Autodesk Fusion 360 part; units mm, degrees
(part 2 of 2)
sketch "Sketch2" plane through (0, 0, 0) normal (0, 0, 1) x (1, 0, 0)
  line L0 (13, -11) -> (-13, -11)
  line L1 (-15, -9) -> (-15, 9)
  line L2 (-13, 11) -> (13, 11)
  line L3 (15, 9) -> (15, -9)
  arc A0 (-13, 11) -> (-15, 9) centre (-13, 9) ccw
  arc A1 (15, 9) -> (13, 11) centre (13, 9) ccw
  arc A2 (13, -11) -> (15, -9) centre (13, -9) ccw
  arc A3 (-15, -9) -> (-13, -11) centre (-13, -9) ccw
  spline S0 degree 3 poles (4.0459, 5.6596) (3.5021, 5.6173) (3.0747, 5.1464) (3.0512, 4.5644) knots 0 0 0 0 1 1 1 1
  line L4 (3.0512, 4.5644) -> (3.04, 4.0279)
  spline S1 degree 3 poles (3.04, 4.0279) (3.0363, 3.6569) (2.7908, 3.3603) (2.4887, 3.3349) knots 0 0 0 0 1 1 1 1
  spline S2 degree 3 poles (2.4887, 3.3349) (2.4646, 3.334) (2.3592, 3.3316) (2.2502, 3.3275) knots 0 0 0 0 1 1 1 1
  spline S3 degree 3 poles (2.2502, 3.3275) (2.1396, 3.3233) (2.0261, 3.3191) (1.9932, 3.3163) knots 0 0 0 0 1 1 1 1
  spline S4 degree 3 poles (1.9932, 3.3163) (1.6944, 3.2927) (1.4246, 3.1392) (1.2406, 2.8953) knots 0 0 0 0 1 1 1 1
  spline S5 degree 3 poles (1.2406, 2.8953) (1.1016, 2.7203) (1.0144, 2.5064) (0.991, 2.2806) knots 0 0 0 0 1 1 1 1
  spline S6 degree 3 poles (0.991, 2.2806) (0.9833, 2.1986) (0.9814, 2.1189) (0.9873, 2.0459) knots 0 0 0 0 1 1 1 1
  spline S7 degree 3 poles (0.9873, 2.0459) (0.9878, 2.0323) (0.9902, 1.9387) (0.991, 1.8522) knots 0 0 0 0 1 1 1 1
  spline S8 degree 2 poles (0.991, 1.8522) (0.9918, 1.7658) (0.991, 1.6846) knots 0 0 0 1 1 1
  spline S9 degree 3 poles (0.991, 1.6846) (0.9873, 1.3122) (0.7435, 1.0171) (0.4322, 0.9916) knots 0 0 0 0 1 1 1 1
  line L5 (0.4322, 0.9916) -> (-0.067, 0.9544)
  spline S10 degree 3 poles (-0.067, 0.9544) (-0.567, 0.9157) (-0.9691, 0.5308) (-1.0431, 0.0267) knots 0 0 0 0 1 1 1 1
  spline S11 degree 3 poles (-1.0431, 0.0267) (-1.0554, -0.0509) (-1.0599, -0.2159) (-1.0617, -0.2489) knots 0 0 0 0 1 1 1 1
  line L6 (-1.0617, -0.2489) -> (-1.0729, -0.7295)
  spline S12 degree 3 poles (-1.0729, -0.7295) (-1.0716, -1.0904) (-1.3155, -1.3812) (-1.6429, -1.4113) knots 0 0 0 0 1 1 1 1
  spline S13 degree 3 poles (-1.6429, -1.4113) (-1.6727, -1.4113) (-1.7757, -1.4076) (-1.8813, -1.4076) knots 0 0 0 0 1 1 1 1
  spline S14 degree 3 poles (-1.8813, -1.4076) (-2.0004, -1.4076) (-2.0851, -1.4106) (-2.1384, -1.4187) knots 0 0 0 0 1 1 1 1
  spline S15 degree 3 poles (-2.1384, -1.4187) (-2.5218, -1.4731) (-2.8335, -1.6981) (-2.9952, -2.026) knots 0 0 0 0 1 1 1 1
  spline S16 degree 3 poles (-2.9952, -2.026) (-3.1043, -2.2305) (-3.153, -2.4605) (-3.1331, -2.6891) knots 0 0 0 0 1 1 1 1
  spline S17 degree 2 poles (-3.1331, -2.6891) (-3.1319, -2.7171) (-3.1219, -3.0766) knots 0 0 0 1 1 1
  spline S18 degree 3 poles (-3.1219, -3.0766) (-3.1164, -3.4412) (-3.3659, -3.729) (-3.6993, -3.7546) knots 0 0 0 0 1 1 1 1
  spline S19 degree 2 poles (-3.6993, -3.7546) (-3.9764, -3.766) (-4.5674, -3.7807) knots 0 0 0 1 1 1
  spline S20 degree 3 poles (-4.5674, -3.7807) (-4.8976, -3.777) (-5.1727, -3.4978) (-5.2044, -3.1287) knots 0 0 0 0 1 1 1 1
  line L7 (-5.2044, -3.1287) -> (-5.2156, -2.9574)
  spline S21 degree 3 poles (-5.2156, -2.9574) (-5.219, -2.9233) (-5.217, -2.8652) (-5.2156, -2.8083) knots 0 0 0 0 1 1 1 1
  spline S22 degree 3 poles (-5.2156, -2.8083) (-5.2156, -2.7383) (-5.2153, -2.6722) (-5.2193, -2.6183) knots 0 0 0 0 1 1 1 1
  spline S23 degree 3 poles (-5.2193, -2.6183) (-5.251, -2.2243) (-5.4718, -1.8745) (-5.8005, -1.687) knots 0 0 0 0 1 1 1 1
  spline S24 degree 3 poles (-5.8005, -1.687) (-5.9946, -1.5677) (-6.223, -1.5137) (-6.4338, -1.5305) knots 0 0 0 0 1 1 1 1
  line L8 (-6.4338, -1.5305) -> (-6.4674, -1.5342)
  spline S25 degree 3 poles (-6.4674, -1.5342) (-6.4962, -1.5355) (-6.5295, -1.536) (-6.553, -1.538) knots 0 0 0 0 1 1 1 1
  line L9 (-6.553, -1.538) -> (-6.7877, -1.5342)
  spline S26 degree 3 poles (-6.7877, -1.5342) (-7.1178, -1.5324) (-7.3917, -1.2536) (-7.4248, -0.8823) knots 0 0 0 0 1 1 1 1
  line L10 (-7.4248, -0.8823) -> (-7.4658, -0.4017)
  spline S27 degree 3 poles (-7.4658, -0.4017) (-7.465, -0.3887) (-7.4643, -0.374) (-7.4658, -0.357) knots 0 0 0 0 1 1 1 1
  spline S28 degree 3 poles (-7.4658, -0.357) (-7.5196, 0.2738) (-8.055, 0.7631) (-8.6542, 0.7159) knots 0 0 0 0 1 1 1 1
  spline S29 degree 3 poles (-8.6542, 0.7159) (-8.9328, 0.6945) (-9.1922, 0.562) (-9.3769, 0.3434) knots 0 0 0 0 1 1 1 1
  spline S30 degree 3 poles (-9.3769, 0.3434) (-9.5782, 0.1068) (-9.6758, -0.2119) (-9.6489, -0.5321) knots 0 0 0 0 1 1 1 1
  spline S31 degree 3 poles (-9.6489, -0.5321) (-9.6, -1.1036) (-9.1563, -1.5632) (-8.6095, -1.6013) knots 0 0 0 0 1 1 1 1
  line L11 (-8.6095, -1.6013) -> (-8.1028, -1.6236)
  spline S32 degree 3 poles (-8.1028, -1.6236) (-7.7639, -1.6346) (-7.4867, -1.9029) (-7.4583, -2.2458) knots 0 0 0 0 1 1 1 1
  line L12 (-7.4583, -2.2458) -> (-7.4397, -2.6481)
  spline S33 degree 3 poles (-7.4397, -2.6481) (-7.4378, -2.6968) (-7.4361, -2.7355) (-7.4322, -2.7785) knots 0 0 0 0 1 1 1 1
  spline S34 degree 3 poles (-7.4322, -2.7785) (-7.4053, -3.0916) (-7.2625, -3.376) (-7.0336, -3.5758) knots 0 0 0 0 1 1 1 1
  spline S35 degree 3 poles (-7.0336, -3.5758) (-6.8658, -3.7313) (-6.6644, -3.8268) (-6.4487, -3.8552) knots 0 0 0 0 1 1 1 1
  spline S36 degree 3 poles (-6.4487, -3.8552) (-6.3703, -3.867) (-6.2961, -3.8702) (-6.214, -3.8664) knots 0 0 0 0 1 1 1 1
  spline S37 degree 2 poles (-6.214, -3.8664) (-6.1486, -3.8664) (-5.8862, -3.8664) knots 0 0 0 1 1 1
  spline S38 degree 3 poles (-5.8862, -3.8664) (-5.5473, -3.8773) (-5.2676, -4.1511) (-5.2379, -4.4997) knots 0 0 0 0 1 1 1 1
  line L13 (-5.2379, -4.4997) -> (-5.1932, -5.0362)
  spline S39 degree 3 poles (-5.1932, -5.0362) (-5.1463, -5.5846) (-4.7415, -6.033) (-4.2283, -6.1016) knots 0 0 0 0 1 1 1 1
  spline S40 degree 3 poles (-4.2283, -6.1016) (-4.1746, -6.1095) (-4.1195, -6.1128) (-4.0682, -6.1128) knots 0 0 0 0 1 1 1 1
  spline S41 degree 3 poles (-4.0682, -6.1128) (-4.0434, -6.1128) (-4.0177, -6.1141) (-3.9936, -6.1128) knots 0 0 0 0 1 1 1 1
  spline S42 degree 3 poles (-3.9936, -6.1128) (-3.4506, -6.0698) (-3.0247, -5.5991) (-3.0027, -5.0175) knots 0 0 0 0 1 1 1 1
  line L14 (-3.0027, -5.0175) -> (-2.9915, -4.4811)
  spline S43 degree 3 poles (-2.9915, -4.4811) (-2.9878, -4.1081) (-2.742, -3.8123) (-2.4364, -3.7881) knots 0 0 0 0 1 1 1 1
  spline S44 degree 2 poles (-2.4364, -3.7881) (-2.3291, -3.7855) (-2.2129, -3.7807) knots 0 0 0 1 1 1
  spline S45 degree 3 poles (-2.2129, -3.7807) (-2.0967, -3.7759) (-1.9752, -3.772) (-1.9446, -3.7695) knots 0 0 0 0 1 1 1 1
  spline S46 degree 3 poles (-1.9446, -3.7695) (-1.6459, -3.7467) (-1.3768, -3.5944) (-1.1921, -3.3523) knots 0 0 0 0 1 1 1 1
  spline S47 degree 3 poles (-1.1921, -3.3523) (-1.0505, -3.1759) (-0.9616, -2.9604) (-0.9387, -2.7338) knots 0 0 0 0 1 1 1 1
  spline S48 degree 3 poles (-0.9387, -2.7338) (-0.931, -2.6518) (-0.9291, -2.5728) (-0.935, -2.4991) knots 0 0 0 0 1 1 1 1
  spline S49 degree 2 poles (-0.935, -2.4991) (-0.935, -2.4638) (-0.9387, -2.1378) knots 0 0 0 1 1 1
  spline S50 degree 3 poles (-0.9387, -2.1378) (-0.9351, -1.7654) (-0.6942, -1.469) (-0.3837, -1.4448) knots 0 0 0 0 1 1 1 1
  line L15 (-0.3837, -1.4448) -> (0.1155, -1.4076)
  spline S51 degree 3 poles (0.1155, -1.4076) (0.6107, -1.3673) (1.018, -0.9888) (1.1065, -0.4911) knots 0 0 0 0 1 1 1 1
  spline S52 degree 3 poles (1.1065, -0.4911) (1.1072, -0.4861) (1.1115, -0.4749) (1.114, -0.4427) knots 0 0 0 0 1 1 1 1
  spline S53 degree 3 poles (1.114, -0.4427) (1.1164, -0.4104) (1.1204, -0.3544) (1.1251, -0.2452) knots 0 0 0 0 1 1 1 1
  line L16 (1.1251, -0.2452) -> (1.1214, 0.2801)
  spline S54 degree 3 poles (1.1214, 0.2801) (1.1196, 0.6442) (1.3699, 0.9362) (1.7026, 0.9618) knots 0 0 0 0 1 1 1 1
  line L17 (1.7026, 0.9618) -> (1.8032, 0.9693)
  line L18 (1.8032, 0.9693) -> (1.8255, 0.9693)
  spline S55 degree 3 poles (1.8255, 0.9693) (1.8551, 0.9693) (1.8984, 0.9656) (1.9447, 0.9656) knots 0 0 0 0 1 1 1 1
  spline S56 degree 3 poles (1.9447, 0.9656) (2.0328, 0.9617) (2.1257, 0.9614) (2.1757, 0.9656) knots 0 0 0 0 1 1 1 1
  spline S57 degree 3 poles (2.1757, 0.9656) (2.5513, 0.9954) (2.8768, 1.2246) (3.0475, 1.5728) knots 0 0 0 0 1 1 1 1
  spline S58 degree 3 poles (3.0475, 1.5728) (3.1445, 1.7584) (3.1892, 1.978) (3.1816, 2.2285) knots 0 0 0 0 1 1 1 1
  spline S59 degree 2 poles (3.1816, 2.2285) (3.1778, 2.3719) (3.1704, 2.6234) knots 0 0 0 1 1 1
  spline S60 degree 3 poles (3.1704, 2.6234) (3.1668, 2.9873) (3.4171, 3.2782) (3.7479, 3.3051) knots 0 0 0 0 1 1 1 1
  spline S61 degree 2 poles (3.7479, 3.3051) (4.4296, 3.3308) (4.6159, 3.3275) knots 0 0 0 1 1 1
  spline S62 degree 3 poles (4.6196, 3.3275) (4.9499, 3.3239) (5.2256, 3.0454) (5.2567, 2.6867) knots 0 0 0 0 1 1 1 1
  spline S63 degree 3 poles (5.2567, 2.6867) (5.2568, 2.6344) (5.2634, 2.2542) (5.2716, 2.1652) knots 0 0 0 0 1 1 1 1
  spline S64 degree 3 poles (5.2716, 2.1652) (5.3046, 1.772) (5.5193, 1.4251) (5.8453, 1.2375) knots 0 0 0 0 1 1 1 1
  spline S65 degree 3 poles (5.8453, 1.2375) (6.0161, 1.1303) (6.2078, 1.0736) (6.4041, 1.0736) knots 0 0 0 0 1 1 1 1
  spline S66 degree 3 poles (6.4041, 1.0736) (6.4302, 1.0736) (6.4563, 1.0749) (6.4786, 1.0773) knots 0 0 0 0 1 1 1 1
  spline S67 degree 3 poles (6.4786, 1.0773) (6.5101, 1.078) (6.838, 1.081) (6.84, 1.081) knots 0 0 0 0 1 1 1 1
  spline S68 degree 3 poles (6.84, 1.081) (7.1717, 1.0774) (7.4446, 0.799) (7.477, 0.4291) knots 0 0 0 0 1 1 1 1
  spline S69 degree 3 poles (7.477, 0.4291) (7.4776, 0.422) (7.5175, -0.0822) (7.518, -0.0962) knots 0 0 0 0 1 1 1 1
  spline S70 degree 3 poles (7.518, -0.0962) (7.5732, -0.7268) (8.1044, -1.219) (8.7065, -1.1691) knots 0 0 0 0 1 1 1 1
  spline S71 degree 3 poles (8.7065, -1.1691) (8.9852, -1.1477) (9.2401, -1.0144) (9.4255, -0.7966) knots 0 0 0 0 1 1 1 1
  spline S72 degree 3 poles (9.4255, -0.7966) (9.6268, -0.5593) (9.7281, -0.2393) (9.7012, 0.0789) knots 0 0 0 0 1 1 1 1
  spline S73 degree 3 poles (9.7012, 0.0789) (9.6521, 0.6503) (9.2049, 1.1107) (8.658, 1.1481) knots 0 0 0 0 1 1 1 1
  line L19 (8.658, 1.1481) -> (8.1588, 1.1705)
  spline S74 degree 3 poles (8.1588, 1.1705) (7.8184, 1.1814) (7.5389, 1.4527) (7.5106, 1.7963) knots 0 0 0 0 1 1 1 1
  spline S75 degree 3 poles (7.5106, 1.7963) (7.5083, 1.8506) (7.4867, 2.2523) (7.4808, 2.3216) knots 0 0 0 0 1 1 1 1
  line L20 (7.4808, 2.3216) -> (7.4808, 2.3253)
  spline S76 degree 3 poles (7.4808, 2.3253) (7.4552, 2.6352) (7.3123, 2.9185) (7.0859, 3.1189) knots 0 0 0 0 1 1 1 1
  spline S77 degree 3 poles (7.0859, 3.1189) (6.9172, 3.2757) (6.7121, 3.3736) (6.4935, 3.402) knots 0 0 0 0 1 1 1 1
  spline S78 degree 3 poles (6.4935, 3.402) (6.4172, 3.4138) (6.3463, 3.419) (6.2626, 3.4132) knots 0 0 0 0 1 1 1 1
  spline S79 degree 3 poles (6.2626, 3.4132) (6.1965, 3.4132) (5.9468, 3.4168) (5.9384, 3.4169) knots 0 0 0 0 1 1 1 1
  line L21 (5.9384, 3.4169) -> (5.9347, 3.4169)
  spline S80 degree 3 poles (5.9347, 3.4169) (5.5958, 3.4294) (5.3192, 3.6983) (5.2902, 4.0465) knots 0 0 0 0 1 1 1 1
  line L22 (5.2902, 4.0465) -> (5.2418, 4.583)
  spline S81 degree 3 poles (5.2418, 4.583) (5.1943, 5.1308) (4.7895, 5.5805) (4.2769, 5.6485) knots 0 0 0 0 1 1 1 1
  spline S82 degree 3 poles (4.2769, 5.6485) (4.1971, 5.6602) (4.1232, 5.6656) (4.0459, 5.6596) knots 0 0 0 0 1 1 1 1
  spline S83 degree 3 poles (2.0453, 7.8949) (1.4432, 7.8459) (0.9839, 7.3052) (0.9761, 6.6394) knots 0 0 0 0 1 1 1 1
  line L23 (0.9761, 6.6394) -> (0.9761, 6.0434)
  spline S84 degree 3 poles (0.9761, 6.0434) (0.9797, 5.6358) (0.7138, 5.3125) (0.3651, 5.2796) knots 0 0 0 0 1 1 1 1
  line L24 (0.3651, 5.2796) -> (0.2608, 5.2796)
  spline S85 degree 3 poles (0.2608, 5.2796) (-0.076, 5.2796) (-0.1303, 5.2736) (-0.149, 5.2722) knots 0 0 0 0 1 1 1 1
  spline S86 degree 3 poles (-0.149, 5.2722) (-0.5528, 5.2397) (-0.9047, 4.9814) (-1.0878, 4.5904) knots 0 0 0 0 1 1 1 1
  spline S87 degree 3 poles (-1.0878, 4.5904) (-1.2021, 4.3647) (-1.2542, 4.1071) (-1.2331, 3.8491) knots 0 0 0 0 1 1 1 1
  spline S88 degree 3 poles (-1.2331, 3.8491) (-1.2325, 3.8453) (-1.2309, 3.8092) (-1.2294, 3.7671) knots 0 0 0 0 1 1 1 1
  spline S89 degree 3 poles (-1.2294, 3.7671) (-1.2279, 3.725) (-1.2232, 3.6732) (-1.2219, 3.6218) knots 0 0 0 0 1 1 1 1
  spline S90 degree 2 poles (-1.2219, 3.6218) (-1.2193, 3.5191) (-1.2182, 3.4206) knots 0 0 0 1 1 1
  spline S91 degree 3 poles (-1.2182, 3.4206) (-1.2146, 3.0094) (-1.4806, 2.6825) (-1.8329, 2.6532) knots 0 0 0 0 1 1 1 1
  spline S92 degree 3 poles (-1.8329, 2.6532) (-2.1688, 2.6347) (-2.7558, 2.6272) (-2.7605, 2.6271) knots 0 0 0 0 1 1 1 1
  spline S93 degree 3 poles (-2.7605, 2.6271) (-3.1154, 2.6313) (-3.4103, 2.9423) (-3.4423, 3.3461) knots 0 0 0 0 1 1 1 1
  spline S94 degree 3 poles (-3.4423, 3.3461) (-3.4432, 3.3696) (-3.4466, 3.4939) (-3.4497, 3.6218) knots 0 0 0 0 1 1 1 1
  spline S95 degree 3 poles (-3.4497, 3.6218) (-3.4528, 3.7497) (-3.4569, 3.8808) (-3.4609, 3.931) knots 0 0 0 0 1 1 1 1
  spline S96 degree 3 poles (-3.4609, 3.931) (-3.4968, 4.3707) (-3.729, 4.7587) (-4.0793, 4.9667) knots 0 0 0 0 1 1 1 1
  spline S97 degree 3 poles (-4.0793, 4.9667) (-4.2616, 5.0859) (-4.4689, 5.1492) (-4.6791, 5.1492) knots 0 0 0 0 1 1 1 1
  spline S98 degree 3 poles (-4.6791, 5.1492) (-4.7098, 5.1492) (-4.7405, 5.1474) (-4.7648, 5.1455) knots 0 0 0 0 1 1 1 1
  spline S99 degree 3 poles (-4.7648, 5.1455) (-4.7791, 5.1448) (-4.8755, 5.1461) (-4.966, 5.1455) knots 0 0 0 0 1 1 1 1
  spline S100 degree 3 poles (-4.966, 5.1455) (-5.0113, 5.1452) (-5.056, 5.1421) (-5.0889, 5.1418) knots 0 0 0 0 1 1 1 1
  spline S101 degree 3 poles (-5.0889, 5.1418) (-5.1054, 5.1417) (-5.1203, 5.1419) (-5.1299, 5.1418) knots 0 0 0 0 1 1 1 1
  spline S102 degree 3 poles (-5.1299, 5.1418) (-5.1347, 5.1417) (-5.1384, 5.1419) (-5.1411, 5.1418) knots 0 0 0 0 1 1 1 1
  line L25 (-5.1411, 5.1418) -> (-5.1448, 5.1418)
  spline S103 degree 3 poles (-5.1448, 5.1418) (-5.4952, 5.1453) (-5.8088, 5.5001) (-5.8415, 5.9167) knots 0 0 0 0 1 1 1 1
  spline S104 degree 2 poles (-5.8415, 5.9167) (-5.8525, 6.059) (-5.8638, 6.2036) knots 0 0 0 1 1 1
  spline S105 degree 3 poles (-5.8638, 6.2036) (-5.8695, 6.2759) (-5.8781, 6.3486) (-5.8825, 6.4047) knots 0 0 0 0 1 1 1 1
  spline S106 degree 3 poles (-5.8825, 6.4047) (-5.8846, 6.4328) (-5.8849, 6.4543) (-5.8862, 6.4718) knots 0 0 0 0 1 1 1 1
  spline S107 degree 3 poles (-5.8862, 6.4718) (-5.8875, 6.4893) (-5.8899, 6.5019) (-5.8899, 6.5016) knots 0 0 0 0 1 1 1 1
  line L26 (-5.8899, 6.5016) -> (-5.8899, 6.5053)
  spline S108 degree 3 poles (-5.8899, 6.5053) (-5.9446, 7.1774) (-6.4653, 7.7049) (-7.0783, 7.7049) knots 0 0 0 0 1 1 1 1
  spline S109 degree 3 poles (-7.0783, 7.7049) (-7.1077, 7.7049) (-7.1364, 7.7069) (-7.1677, 7.7049) knots 0 0 0 0 1 1 1 1
  spline S110 degree 3 poles (-7.1677, 7.7049) (-7.4614, 7.6808) (-7.733, 7.5349) (-7.9315, 7.2988) knots 0 0 0 0 1 1 1 1
  spline S111 degree 3 poles (-7.9315, 7.2988) (-8.1548, 7.034) (-8.2617, 6.6735) (-8.2332, 6.3116) knots 0 0 0 0 1 1 1 1
  spline S112 degree 3 poles (-8.2332, 6.3116) (-8.1807, 5.673) (-7.7048, 5.1609) (-7.1156, 5.1194) knots 0 0 0 0 1 1 1 1
  line L27 (-7.1156, 5.1194) -> (-6.5754, 5.0934)
  spline S113 degree 3 poles (-6.5754, 5.0934) (-6.2178, 5.0815) (-5.8993, 4.7373) (-5.8676, 4.352) knots 0 0 0 0 1 1 1 1
  spline S114 degree 3 poles (-5.8676, 4.352) (-5.8661, 4.2932) (-5.8402, 3.832) (-5.834, 3.7597) knots 0 0 0 0 1 1 1 1
  spline S115 degree 3 poles (-5.834, 3.7597) (-5.8055, 3.4129) (-5.6588, 3.0933) (-5.4168, 2.8693) knots 0 0 0 0 1 1 1 1
  spline S116 degree 3 poles (-5.4168, 2.8693) (-5.2351, 2.6943) (-5.0153, 2.5858) (-4.7834, 2.5526) knots 0 0 0 0 1 1 1 1
  spline S117 degree 3 poles (-4.7834, 2.5526) (-4.7472, 2.5463) (-4.7035, 2.5452) (-4.6456, 2.5452) knots 0 0 0 0 1 1 1 1
  spline S118 degree 3 poles (-4.6456, 2.5452) (-4.6038, 2.5452) (-4.5356, 2.5432) (-4.4929, 2.5452) knots 0 0 0 0 1 1 1 1
  line L28 (-4.4929, 2.5452) -> (-4.1799, 2.5414)
  spline S119 degree 3 poles (-4.1799, 2.5414) (-3.8186, 2.5267) (-3.5196, 2.2229) (-3.487, 1.8299) knots 0 0 0 0 1 1 1 1
  line L29 (-3.487, 1.8299) -> (-3.4385, 1.2263)
  spline S120 degree 3 poles (-3.4385, 1.2263) (-3.3876, 0.615) (-2.9511, 0.1141) (-2.3991, 0.0379) knots 0 0 0 0 1 1 1 1
  spline S121 degree 3 poles (-2.3991, 0.0379) (-2.3406, 0.028) (-2.2843, 0.0267) (-2.2315, 0.0267) knots 0 0 0 0 1 1 1 1
  spline S122 degree 3 poles (-2.2315, 0.0267) (-2.2044, 0.0267) (-2.1774, 0.0247) (-2.1495, 0.0267) knots 0 0 0 0 1 1 1 1
  spline S123 degree 3 poles (-2.1495, 0.0267) (-1.5651, 0.0743) (-1.1082, 0.5978) (-1.0803, 1.245) knots 0 0 0 0 1 1 1 1
  line L30 (-1.0803, 1.245) -> (-1.0803, 1.2487)
  line L31 (-1.0803, 1.2487) -> (-1.0691, 1.8522)
  spline S124 degree 3 poles (-1.0691, 1.8522) (-1.0641, 2.2718) (-0.8083, 2.6015) (-0.4843, 2.6271) knots 0 0 0 0 1 1 1 1
  spline S125 degree 3 poles (-0.4843, 2.6271) (-0.4617, 2.6285) (-0.3418, 2.633) (-0.2235, 2.6383) knots 0 0 0 0 1 1 1 1
  spline S126 degree 3 poles (-0.2235, 2.6383) (-0.1051, 2.6436) (0.0114, 2.6499) (0.0448, 2.6532) knots 0 0 0 0 1 1 1 1
  spline S127 degree 3 poles (0.0448, 2.6532) (0.3683, 2.6796) (0.6563, 2.8462) (0.8569, 3.1189) knots 0 0 0 0 1 1 1 1
  spline S128 degree 3 poles (0.8569, 3.1189) (1.0071, 3.3149) (1.1019, 3.5507) (1.1251, 3.8006) knots 0 0 0 0 1 1 1 1
  spline S129 degree 3 poles (1.1251, 3.8006) (1.1349, 3.8932) (1.1347, 3.9848) (1.1289, 4.0689) knots 0 0 0 0 1 1 1 1
  spline S130 degree 3 poles (1.1289, 4.0689) (1.1281, 4.0856) (1.1263, 4.1922) (1.1251, 4.2887) knots 0 0 0 0 1 1 1 1
  spline S131 degree 2 poles (1.1251, 4.2887) (1.1239, 4.3852) (1.1251, 4.4749) knots 0 0 0 1 1 1
  spline S132 degree 3 poles (1.1251, 4.4749) (1.1308, 4.8938) (1.3893, 5.225) (1.7212, 5.2536) knots 0 0 0 0 1 1 1 1
  line L32 (1.7212, 5.2536) -> (2.254, 5.2945)
  spline S133 degree 3 poles (2.254, 5.2945) (2.8198, 5.3406) (3.2647, 5.8229) (3.3194, 6.4345) knots 0 0 0 0 1 1 1 1
  spline S134 degree 3 poles (3.3194, 6.4345) (3.3292, 6.5215) (3.331, 6.6109) (3.3232, 6.699) knots 0 0 0 0 1 1 1 1
  spline S135 degree 3 poles (3.3232, 6.699) (3.2647, 7.4027) (2.6924, 7.9493) (2.0453, 7.8949) knots 0 0 0 0 1 1 1 1
  spline S136 degree 3 poles (-8.8405, 5.2573) (-9.3781, 5.2128) (-9.8036, 4.7297) (-9.8277, 4.1359) knots 0 0 0 0 1 1 1 1
  line L33 (-9.8277, 4.1359) -> (-9.8389, 3.5808)
  spline S137 degree 3 poles (-9.8389, 3.5808) (-9.8426, 3.1977) (-10.0794, 2.8977) (-10.3754, 2.873) knots 0 0 0 0 1 1 1 1
  spline S138 degree 3 poles (-10.3754, 2.873) (-10.3996, 2.8722) (-10.5027, 2.8698) (-10.6101, 2.8655) knots 0 0 0 0 1 1 1 1
  spline S139 degree 3 poles (-10.6101, 2.8655) (-10.7192, 2.8612) (-10.8305, 2.8538) (-10.8634, 2.8506) knots 0 0 0 0 1 1 1 1
  spline S140 degree 3 poles (-10.8634, 2.8506) (-11.16, 2.8255) (-11.4279, 2.6707) (-11.6122, 2.4222) knots 0 0 0 0 1 1 1 1
  spline S141 degree 3 poles (-11.6122, 2.4222) (-11.7505, 2.2413) (-11.8367, 2.0206) (-11.8581, 1.7889) knots 0 0 0 0 1 1 1 1
  spline S142 degree 3 poles (-11.8581, 1.7889) (-11.868, 1.7102) (-11.8676, 1.627) (-11.8618, 1.543) knots 0 0 0 0 1 1 1 1
  spline S143 degree 3 poles (-11.8618, 1.543) (-11.8087, 0.896) (-11.2812, 0.3954) (-10.6808, 0.444) knots 0 0 0 0 1 1 1 1
  spline S144 degree 3 poles (-10.6808, 0.444) (-10.3068, 0.4739) (-9.9812, 0.7117) (-9.8128, 1.0699) knots 0 0 0 0 1 1 1 1
  spline S145 degree 3 poles (-9.8128, 1.0699) (-9.7066, 1.2783) (-9.6601, 1.5123) (-9.6787, 1.7479) knots 0 0 0 0 1 1 1 1
  spline S146 degree 3 poles (-9.6787, 1.7479) (-9.6795, 1.7614) (-9.684, 1.8653) (-9.6861, 1.9603) knots 0 0 0 0 1 1 1 1
  spline S147 degree 2 poles (-9.6861, 1.9603) (-9.6883, 2.0552) (-9.6899, 2.1428) knots 0 0 0 1 1 1
  spline S148 degree 3 poles (-9.6899, 2.1428) (-9.6936, 2.5176) (-9.4519, 2.817) (-9.1273, 2.8432) knots 0 0 0 0 1 1 1 1
  spline S149 degree 2 poles (-9.1273, 2.8432) (-8.6249, 2.8668) (-8.2742, 2.8655) knots 0 0 0 1 1 1
  spline S150 degree 3 poles (-8.2742, 2.8655) (-8.2732, 2.8655) (-8.2715, 2.8656) (-8.2705, 2.8655) knots 0 0 0 0 1 1 1 1
  spline S151 degree 3 poles (-8.2705, 2.8655) (-8.1132, 2.8626) (-7.9448, 2.7694) (-7.8122, 2.6271) knots 0 0 0 0 1 1 1 1
  spline S152 degree 3 poles (-7.8122, 2.6271) (-7.6788, 2.4839) (-7.5815, 2.292) (-7.5663, 2.1093) knots 0 0 0 0 1 1 1 1
  spline S153 degree 3 poles (-7.5663, 2.1093) (-7.5657, 2.0853) (-7.5653, 1.9752) (-7.5626, 1.8597) knots 0 0 0 0 1 1 1 1
  spline S154 degree 3 poles (-7.5626, 1.8597) (-7.5599, 1.7425) (-7.5556, 1.623) (-7.5515, 1.5765) knots 0 0 0 0 1 1 1 1
  spline S155 degree 3 poles (-7.5515, 1.5765) (-7.5186, 1.1754) (-7.3036, 0.8203) (-6.9815, 0.6265) knots 0 0 0 0 1 1 1 1
  spline S156 degree 3 poles (-6.9815, 0.6265) (-6.8132, 0.5172) (-6.6178, 0.4589) (-6.4226, 0.4589) knots 0 0 0 0 1 1 1 1
  spline S157 degree 3 poles (-6.4226, 0.4589) (-6.3954, 0.4589) (-6.3703, 0.4602) (-6.3481, 0.4626) knots 0 0 0 0 1 1 1 1
  spline S158 degree 3 poles (-6.3481, 0.4626) (-6.3159, 0.4632) (-6.0045, 0.4663) (-5.9979, 0.4663) knots 0 0 0 0 1 1 1 1
  spline S159 degree 3 poles (-5.9979, 0.4663) (-5.6758, 0.4627) (-5.407, 0.1757) (-5.3758, -0.2042) knots 0 0 0 0 1 1 1 1
  spline S160 degree 3 poles (-5.3758, -0.2042) (-5.3755, -0.2078) (-5.3634, -0.3287) (-5.3534, -0.4576) knots 0 0 0 0 1 1 1 1
  spline S161 degree 3 poles (-5.3534, -0.4576) (-5.3484, -0.5229) (-5.3462, -0.5915) (-5.3423, -0.6438) knots 0 0 0 0 1 1 1 1
  spline S162 degree 3 poles (-5.3423, -0.6438) (-5.3383, -0.6962) (-5.335, -0.7347) (-5.3348, -0.7407) knots 0 0 0 0 1 1 1 1
  line L34 (-5.3348, -0.7407) -> (-5.3348, -0.7444)
  spline S163 degree 3 poles (-5.3348, -0.7444) (-5.2803, -1.3912) (-4.7562, -1.8927) (-4.1538, -1.8434) knots 0 0 0 0 1 1 1 1
  spline S164 degree 3 poles (-4.1538, -1.8434) (-3.553, -1.7943) (-3.1129, -1.2185) (-3.1666, -0.5656) knots 0 0 0 0 1 1 1 1
  spline S165 degree 3 poles (-3.1666, -0.5656) (-3.2141, 0.0208) (-3.654, 0.4908) (-4.1985, 0.5297) knots 0 0 0 0 1 1 1 1
  line L35 (-4.1985, 0.5297) -> (-4.694, 0.5558)
  spline S166 degree 3 poles (-4.694, 0.5558) (-5.0221, 0.5666) (-5.2956, 0.8434) (-5.3274, 1.1928) knots 0 0 0 0 1 1 1 1
  spline S167 degree 3 poles (-5.3274, 1.1928) (-5.3288, 1.2464) (-5.3521, 1.6713) (-5.3572, 1.7367) knots 0 0 0 0 1 1 1 1
  spline S168 degree 3 poles (-5.3572, 1.7367) (-5.3841, 2.0548) (-5.5222, 2.346) (-5.7446, 2.5526) knots 0 0 0 0 1 1 1 1
  spline S169 degree 3 poles (-5.7446, 2.5526) (-5.9109, 2.7133) (-6.113, 2.8165) (-6.3258, 2.8469) knots 0 0 0 0 1 1 1 1
  line L36 (-6.3258, 2.8469) -> (-6.3295, 2.8469)
  spline S170 degree 3 poles (-6.3295, 2.8469) (-6.4068, 2.8581) (-6.4908, 2.8599) (-6.5568, 2.8544) knots 0 0 0 0 1 1 1 1
  line L37 (-6.5568, 2.8544) -> (-6.5866, 2.8544)
  spline S171 degree 3 poles (-6.5866, 2.8544) (-6.672, 2.8544) (-6.8763, 2.8581) (-6.8846, 2.8581) knots 0 0 0 0 1 1 1 1
  line L38 (-6.8846, 2.8581) -> (-6.8883, 2.8581)
  spline S172 degree 3 poles (-6.8883, 2.8581) (-7.0501, 2.8654) (-7.2235, 2.9601) (-7.3577, 3.1002) knots 0 0 0 0 1 1 1 1
  spline S173 degree 3 poles (-7.3577, 3.1002) (-7.4928, 3.2413) (-7.5889, 3.4252) (-7.6036, 3.6032) knots 0 0 0 0 1 1 1 1
  line L39 (-7.6036, 3.6032) -> (-7.6483, 4.1546)
  spline S174 degree 3 poles (-7.6483, 4.1546) (-7.6938, 4.7167) (-8.0972, 5.1797) (-8.6095, 5.2498) knots 0 0 0 0 1 1 1 1
  spline S175 degree 3 poles (-8.6095, 5.2498) (-8.6609, 5.2578) (-8.7092, 5.2573) (-8.7585, 5.2573) knots 0 0 0 0 1 1 1 1
  spline S176 degree 3 poles (-8.7585, 5.2573) (-8.7841, 5.2573) (-8.8115, 5.2593) (-8.8405, 5.2573) knots 0 0 0 0 1 1 1 1
  spline S177 degree 3 poles (2.2689, -0.8078) (2.2428, -0.8078) (2.2159, -0.8102) (2.1906, -0.8115) knots 0 0 0 0 1 1 1 1
  spline S178 degree 3 poles (2.1906, -0.8115) (1.653, -0.856) (1.2349, -1.3378) (1.2108, -1.9329) knots 0 0 0 0 1 1 1 1
  line L40 (1.2108, -1.9329) -> (1.1997, -2.4879)
  spline S179 degree 3 poles (1.1997, -2.4879) (1.196, -2.8718) (0.956, -3.1717) (0.6595, -3.1958) knots 0 0 0 0 1 1 1 1
  spline S180 degree 3 poles (0.6595, -3.1958) (0.6115, -3.1979) (0.2381, -3.2171) (0.1789, -3.2219) knots 0 0 0 0 1 1 1 1
  spline S181 degree 3 poles (0.1789, -3.2219) (-0.1188, -3.2449) (-0.3855, -3.3996) (-0.57, -3.6503) knots 0 0 0 0 1 1 1 1
  spline S182 degree 3 poles (-0.57, -3.6503) (-0.7061, -3.83) (-0.7932, -4.0471) (-0.8158, -4.2762) knots 0 0 0 0 1 1 1 1
  spline S183 degree 3 poles (-0.8158, -4.2762) (-0.8256, -4.3615) (-0.8275, -4.447) (-0.8195, -4.5258) knots 0 0 0 0 1 1 1 1
  spline S184 degree 3 poles (-0.8195, -4.5258) (-0.819, -4.5436) (-0.8166, -4.6362) (-0.8158, -4.7232) knots 0 0 0 0 1 1 1 1
  spline S185 degree 2 poles (-0.8158, -4.7232) (-0.815, -4.8119) (-0.8158, -4.8946) knots 0 0 0 1 1 1
  spline S186 degree 3 poles (-0.8158, -4.8946) (-0.8195, -5.2778) (-1.0567, -5.5808) (-1.3597, -5.6062) knots 0 0 0 0 1 1 1 1
  line L41 (-1.3597, -5.6062) -> (-1.8515, -5.6471)
  spline S187 degree 3 poles (-1.8515, -5.6471) (-2.3708, -5.6895) (-2.7817, -6.1316) (-2.8313, -6.694) knots 0 0 0 0 1 1 1 1
  spline S188 degree 3 poles (-2.8313, -6.694) (-2.8411, -6.7745) (-2.8408, -6.856) (-2.835, -6.9361) knots 0 0 0 0 1 1 1 1
  spline S189 degree 3 poles (-2.835, -6.9361) (-2.7819, -7.5838) (-2.253, -8.0845) (-1.6578, -8.0352) knots 0 0 0 0 1 1 1 1
  spline S190 degree 3 poles (-1.6578, -8.0352) (-1.1039, -7.9901) (-0.6811, -7.4929) (-0.6743, -6.8803) knots 0 0 0 0 1 1 1 1
  line L42 (-0.6743, -6.8803) -> (-0.6705, -6.3364)
  spline S191 degree 3 poles (-0.6705, -6.3364) (-0.6742, -5.9628) (-0.4352, -5.6653) (-0.1154, -5.636) knots 0 0 0 0 1 1 1 1
  line L43 (-0.1154, -5.636) -> (-0.0186, -5.636)
  spline S192 degree 3 poles (-0.0186, -5.636) (0.2905, -5.636) (0.3435, -5.6322) (0.354, -5.6322) knots 0 0 0 0 1 1 1 1
  line L44 (0.354, -5.6322) -> (0.3577, -5.6322)
  spline S193 degree 3 poles (0.3577, -5.6322) (0.728, -5.6019) (1.0505, -5.3624) (1.2183, -5.0064) knots 0 0 0 0 1 1 1 1
  spline S194 degree 3 poles (1.2183, -5.0064) (1.3245, -4.798) (1.3709, -4.5591) (1.3524, -4.3209) knots 0 0 0 0 1 1 1 1
  spline S195 degree 3 poles (1.3524, -4.3209) (1.3519, -4.3162) (1.3497, -4.285) (1.3487, -4.2464) knots 0 0 0 0 1 1 1 1
  spline S196 degree 3 poles (1.3487, -4.2464) (1.3476, -4.2077) (1.3496, -4.1594) (1.3487, -4.1122) knots 0 0 0 0 1 1 1 1
  spline S197 degree 2 poles (1.3487, -4.1122) (1.3467, -4.0179) (1.3449, -3.9297) knots 0 0 0 1 1 1
  spline S198 degree 3 poles (1.3449, -3.9297) (1.3413, -3.5549) (1.5814, -3.2555) (1.9038, -3.2293) knots 0 0 0 0 1 1 1 1
  line L45 (1.9038, -3.2293) -> (1.9075, -3.2293)
  spline S199 degree 2 poles (1.9075, -3.2293) (2.1786, -3.1985) (2.7569, -3.2032) knots 0 0 0 1 1 1
  spline S200 degree 3 poles (2.7569, -3.2032) (3.0789, -3.2069) (3.3485, -3.4932) (3.379, -3.8626) knots 0 0 0 0 1 1 1 1
  spline S201 degree 3 poles (3.379, -3.8626) (3.3797, -3.8839) (3.3806, -3.9948) (3.3828, -4.1122) knots 0 0 0 0 1 1 1 1
  spline S202 degree 3 poles (3.3828, -4.1122) (3.385, -4.2297) (3.3898, -4.3521) (3.3939, -4.3991) knots 0 0 0 0 1 1 1 1
  spline S203 degree 3 poles (3.3939, -4.3991) (3.427, -4.8027) (3.6394, -5.1616) (3.9602, -5.3528) knots 0 0 0 0 1 1 1 1
  spline S204 degree 3 poles (3.9602, -5.3528) (4.1291, -5.4621) (4.3208, -5.5205) (4.5153, -5.5205) knots 0 0 0 0 1 1 1 1
  spline S205 degree 3 poles (4.5153, -5.5205) (4.5401, -5.5205) (4.5676, -5.518) (4.5898, -5.5167) knots 0 0 0 0 1 1 1 1
  spline S206 degree 3 poles (4.5898, -5.5167) (4.603, -5.5161) (4.6929, -5.5137) (4.7761, -5.513) knots 0 0 0 0 1 1 1 1
  spline S207 degree 2 poles (4.7761, -5.513) (4.8593, -5.5123) (4.94, -5.513) knots 0 0 0 1 1 1
  spline S208 degree 3 poles (4.94, -5.513) (5.2595, -5.5148) (5.5721, -5.8335) (5.6031, -6.2134) knots 0 0 0 0 1 1 1 1
  spline S209 degree 2 poles (5.6031, -6.2134) (5.6151, -6.3415) (5.6255, -6.4742) knots 0 0 0 1 1 1
  spline S210 degree 3 poles (5.6255, -6.4742) (5.6359, -6.6069) (5.6437, -6.7468) (5.6441, -6.7536) knots 0 0 0 0 1 1 1 1
  spline S211 degree 3 poles (5.6441, -6.7536) (5.6951, -7.3715) (6.1761, -7.8563) (6.7394, -7.8563) knots 0 0 0 0 1 1 1 1
  spline S212 degree 3 poles (6.7394, -7.8563) (6.7668, -7.8563) (6.7937, -7.8551) (6.8214, -7.8526) knots 0 0 0 0 1 1 1 1
  spline S213 degree 3 poles (6.8214, -7.8526) (7.0927, -7.8298) (7.3423, -7.6971) (7.5255, -7.4801) knots 0 0 0 0 1 1 1 1
  spline S214 degree 3 poles (7.5255, -7.4801) (7.7302, -7.2366) (7.8325, -6.9076) (7.8049, -6.5748) knots 0 0 0 0 1 1 1 1
  spline S215 degree 3 poles (7.8049, -6.5748) (7.7567, -5.9877) (7.3157, -5.5132) (6.7729, -5.4758) knots 0 0 0 0 1 1 1 1
  line L46 (6.7729, -5.4758) -> (6.2775, -5.4534)
  spline S216 degree 3 poles (6.2775, -5.4534) (5.9491, -5.4426) (5.6352, -5.1345) (5.6069, -4.7828) knots 0 0 0 0 1 1 1 1
  spline S217 degree 3 poles (5.6069, -4.7828) (5.6049, -4.731) (5.5821, -4.3052) (5.5771, -4.2389) knots 0 0 0 0 1 1 1 1
  line L47 (5.5771, -4.2389) -> (5.5771, -4.2352)
  spline S218 degree 3 poles (5.5771, -4.2352) (5.5501, -3.9172) (5.4123, -3.6284) (5.1896, -3.423) knots 0 0 0 0 1 1 1 1
  spline S219 degree 3 poles (5.1896, -3.423) (5.0225, -3.2616) (4.821, -3.1593) (4.6084, -3.1287) knots 0 0 0 0 1 1 1 1
  spline S220 degree 3 poles (4.6084, -3.1287) (4.5779, -3.1248) (4.5346, -3.1213) (4.4818, -3.1213) knots 0 0 0 0 1 1 1 1
  spline S221 degree 3 poles (4.4818, -3.1213) (4.4424, -3.1213) (4.3817, -3.1231) (4.3439, -3.125) knots 0 0 0 0 1 1 1 1
  line L48 (4.3439, -3.125) -> (4.0534, -3.1138)
  spline S222 degree 3 poles (4.0534, -3.1138) (3.7225, -3.1011) (3.4529, -2.8243) (3.4237, -2.4656) knots 0 0 0 0 1 1 1 1
  line L49 (3.4237, -2.4656) -> (3.379, -1.9142)
  spline S223 degree 3 poles (3.379, -1.9142) (3.3331, -1.3535) (2.9305, -0.8954) (2.4253, -0.8227) knots 0 0 0 0 1 1 1 1
  spline S224 degree 3 poles (2.4253, -0.8227) (2.3707, -0.8126) (2.3173, -0.8078) (2.2689, -0.8078) knots 0 0 0 0 1 1 1 1
  spline S225 degree 3 poles (4.1837, 1.3307) (3.5909, 1.282) (3.154, 0.7104) (3.2077, 0.0603) knots 0 0 0 0 1 1 1 1
  spline S226 degree 3 poles (3.2077, 0.0603) (3.2532, -0.5222) (3.6891, -0.9925) (4.2285, -1.0313) knots 0 0 0 0 1 1 1 1
  line L50 (4.2285, -1.0313) -> (4.7202, -1.0574)
  spline S227 degree 3 poles (4.7202, -1.0574) (5.0476, -1.0689) (5.3182, -1.3427) (5.3461, -1.6944) knots 0 0 0 0 1 1 1 1
  spline S228 degree 3 poles (5.3461, -1.6944) (5.3483, -1.745) (5.3682, -2.1723) (5.3722, -2.2346) knots 0 0 0 0 1 1 1 1
  spline S229 degree 3 poles (5.3722, -2.2346) (5.3982, -2.549) (5.5369, -2.8374) (5.7559, -3.043) knots 0 0 0 0 1 1 1 1
  spline S230 degree 3 poles (5.7559, -3.043) (5.7567, -3.0439) (5.7588, -3.0422) (5.7596, -3.043) knots 0 0 0 0 1 1 1 1
  spline S231 degree 3 poles (5.7596, -3.043) (5.7604, -3.0438) (5.7588, -3.046) (5.7596, -3.0468) knots 0 0 0 0 1 1 1 1
  spline S232 degree 3 poles (5.7596, -3.0468) (5.924, -3.2056) (6.1268, -3.3071) (6.3371, -3.3374) knots 0 0 0 0 1 1 1 1
  spline S233 degree 3 poles (6.3371, -3.3374) (6.415, -3.3485) (6.4972, -3.3546) (6.5643, -3.3485) knots 0 0 0 0 1 1 1 1
  line L51 (6.5643, -3.3485) -> (6.5904, -3.3485)
  spline S234 degree 3 poles (6.5904, -3.3485) (6.6762, -3.3485) (6.8883, -3.3485) (6.8922, -3.3485) knots 0 0 0 0 1 1 1 1
  spline S235 degree 3 poles (6.8922, -3.3485) (7.0508, -3.3556) (7.2212, -3.4512) (7.3541, -3.5907) knots 0 0 0 0 1 1 1 1
  spline S236 degree 3 poles (7.3541, -3.5907) (7.4879, -3.731) (7.5818, -3.9129) (7.5963, -4.0899) knots 0 0 0 0 1 1 1 1
  line L52 (7.5963, -4.0899) -> (7.641, -4.6413)
  spline S237 degree 3 poles (7.641, -4.6413) (7.6878, -5.2007) (8.0889, -5.6596) (8.5947, -5.7291) knots 0 0 0 0 1 1 1 1
  spline S238 degree 3 poles (8.5947, -5.7291) (8.6445, -5.7349) (8.6957, -5.7366) (8.7437, -5.7366) knots 0 0 0 0 1 1 1 1
  spline S239 degree 3 poles (8.7437, -5.7366) (8.7715, -5.7366) (8.7964, -5.7347) (8.8219, -5.7328) knots 0 0 0 0 1 1 1 1
  spline S240 degree 3 poles (8.8219, -5.7328) (9.3556, -5.6897) (9.7746, -5.2106) (9.798, -4.6189) knots 0 0 0 0 1 1 1 1
  line L53 (9.798, -4.6189) -> (9.8092, -4.0675)
  spline S241 degree 3 poles (9.8092, -4.0675) (9.8131, -3.6863) (10.0488, -3.3874) (10.3419, -3.3634) knots 0 0 0 0 1 1 1 1
  spline S242 degree 3 poles (10.3419, -3.3634) (10.3922, -3.3618) (10.7619, -3.3451) (10.8225, -3.3411) knots 0 0 0 0 1 1 1 1
  line L54 (10.8225, -3.3411) -> (10.8262, -3.3411)
  spline S243 degree 3 poles (10.8262, -3.3411) (11.1212, -3.3161) (11.3845, -3.1641) (11.5676, -2.9127) knots 0 0 0 0 1 1 1 1
  spline S244 degree 3 poles (11.5676, -2.9127) (11.7051, -2.7329) (11.7885, -2.5134) (11.8098, -2.283) knots 0 0 0 0 1 1 1 1
  spline S245 degree 3 poles (11.8098, -2.283) (11.8175, -2.2052) (11.8214, -2.1251) (11.8135, -2.0409) knots 0 0 0 0 1 1 1 1
  spline S246 degree 3 poles (11.8135, -2.0409) (11.7618, -1.396) (11.2411, -0.8978) (10.6474, -0.9456) knots 0 0 0 0 1 1 1 1
  spline S247 degree 3 poles (10.6474, -0.9456) (10.2774, -0.9762) (9.9539, -1.211) (9.7868, -1.5678) knots 0 0 0 0 1 1 1 1
  spline S248 degree 3 poles (9.7868, -1.5678) (9.6807, -1.7754) (9.6332, -2.0107) (9.6527, -2.2458) knots 0 0 0 0 1 1 1 1
  spline S249 degree 3 poles (9.6527, -2.2458) (9.6535, -2.2593) (9.658, -2.36) (9.6602, -2.4544) knots 0 0 0 0 1 1 1 1
  spline S250 degree 2 poles (9.6602, -2.4544) (9.6623, -2.5489) (9.6639, -2.637) knots 0 0 0 1 1 1
  spline S251 degree 3 poles (9.6639, -2.637) (9.6691, -3.0097) (9.4276, -3.3081) (9.1051, -3.3336) knots 0 0 0 0 1 1 1 1
  spline S252 degree 2 poles (9.1051, -3.3336) (8.8757, -3.347) (8.2594, -3.3597) knots 0 0 0 1 1 1
  spline S253 degree 3 poles (8.2594, -3.3597) (8.1037, -3.3578) (7.937, -3.2637) (7.8049, -3.1213) knots 0 0 0 0 1 1 1 1
  spline S254 degree 3 poles (7.8049, -3.1213) (7.6735, -2.9797) (7.579, -2.7917) (7.5627, -2.6109) knots 0 0 0 0 1 1 1 1
  spline S255 degree 3 poles (7.5627, -2.6109) (7.5627, -2.5617) (7.556, -2.1665) (7.5478, -2.0744) knots 0 0 0 0 1 1 1 1
  spline S256 degree 3 poles (7.5478, -2.0744) (7.5155, -1.6735) (7.3008, -1.3207) (6.9816, -1.1282) knots 0 0 0 0 1 1 1 1
  spline S257 degree 3 poles (6.9816, -1.1282) (6.8134, -1.0201) (6.6234, -0.9605) (6.4302, -0.9605) knots 0 0 0 0 1 1 1 1
  spline S258 degree 3 poles (6.4302, -0.9605) (6.4031, -0.9605) (6.377, -0.9623) (6.3557, -0.9642) knots 0 0 0 0 1 1 1 1
  spline S259 degree 3 poles (6.3557, -0.9642) (6.324, -0.9648) (6.0158, -0.9679) (6.0092, -0.968) knots 0 0 0 0 1 1 1 1
  spline S260 degree 3 poles (6.0092, -0.968) (5.6921, -0.9654) (5.4227, -0.6797) (5.3908, -0.3011) knots 0 0 0 0 1 1 1 1
  spline S261 degree 2 poles (5.3908, -0.3011) (5.3821, -0.1778) (5.3722, -0.0478) knots 0 0 0 1 1 1
  spline S262 degree 3 poles (5.3722, -0.0478) (5.3672, 0.0173) (5.3611, 0.0828) (5.3573, 0.1348) knots 0 0 0 0 1 1 1 1
  spline S263 degree 3 poles (5.3573, 0.1348) (5.3534, 0.1868) (5.35, 0.2295) (5.3498, 0.2354) knots 0 0 0 0 1 1 1 1
  spline S264 degree 3 poles (5.3498, 0.2354) (5.2968, 0.8794) (4.7808, 1.3799) (4.1837, 1.3307) knots 0 0 0 0 1 1 1 1
  spline S265 degree 3 poles (-13.0651, 0.0044) (-13.0939, 0.0044) (-13.1195, 0.004) (-13.1471, 0.0007) knots 0 0 0 0 1 1 1 1
  spline S266 degree 3 poles (-13.1471, 0.0007) (-13.752, -0.0465) (-14.1993, -0.6046) (-14.1455, -1.2399) knots 0 0 0 0 1 1 1 1
  spline S267 degree 3 poles (-14.1455, -1.2399) (-14.0924, -1.8692) (-13.5632, -2.3562) (-12.9497, -2.3091) knots 0 0 0 0 1 1 1 1
  spline S268 degree 3 poles (-12.9497, -2.3091) (-12.654, -2.2856) (-12.3864, -2.1384) (-12.1971, -1.8993) knots 0 0 0 0 1 1 1 1
  spline S269 degree 3 poles (-12.1971, -1.8993) (-12.0147, -1.6664) (-11.9257, -1.3728) (-11.9512, -1.0685) knots 0 0 0 0 1 1 1 1
  spline S270 degree 3 poles (-11.9512, -1.0685) (-12.0031, -0.4675) (-12.4926, 0.0044) (-13.0651, 0.0044) knots 0 0 0 0 1 1 1 1
  spline S271 degree 3 poles (13.0466, 1.7926) (13.0198, 1.7926) (12.9934, 1.7922) (12.9647, 1.7889) knots 0 0 0 0 1 1 1 1
  spline S272 degree 3 poles (12.9647, 1.7889) (12.3591, 1.7418) (11.9124, 1.1836) (11.9662, 0.5483) knots 0 0 0 0 1 1 1 1
  spline S273 degree 3 poles (11.9662, 0.5483) (12.0194, -0.0809) (12.5492, -0.568) (13.1621, -0.5209) knots 0 0 0 0 1 1 1 1
  spline S274 degree 3 poles (13.1621, -0.5209) (13.4586, -0.4981) (13.726, -0.3496) (13.9146, -0.1111) knots 0 0 0 0 1 1 1 1
  spline S275 degree 3 poles (13.9146, -0.1111) (14.0985, 0.1219) (14.186, 0.4156) (14.1605, 0.7197) knots 0 0 0 0 1 1 1 1
  spline S276 degree 3 poles (14.1605, 0.7197) (14.1108, 1.3202) (13.6205, 1.7926) (13.0466, 1.7926) knots 0 0 0 0 1 1 1 1
  line L55 (4.6159, 3.3275) -> (4.6196, 3.3275)
  point P0 (-15, -11)
  point P1 (-15, 11)
  point P2 (15, 11)
  dimension "d7" = 30
  dimension "d8" = 22
  dimension "d9" = 2
  dimension "d10" = 2
  dimension "d11" = 2
  dimension "d12" = 2
  constraint horizontal L0
  constraint perpendicular L0 L1
  constraint parallel L0 L2
  constraint parallel L1 L3
  constraint coincident P1 L1
  constraint coincident P1 L2
  constraint tangent L1 A0
  constraint tangent L2 A0
  constraint coincident P2 L2
  constraint coincident P2 L3
  constraint tangent L2 A1
  constraint tangent L3 A1
  constraint tangent L0 A2
  constraint tangent L3 A2
  constraint coincident P0 L0
  constraint coincident P0 L1
  constraint tangent L0 A3
  constraint tangent L1 A3
  constraint horizontal L55
  measures "d7" distance of P1 P2
  measures "d8" distance of P0 P1
  measures "d9" radius of A0
  measures "d10" radius of A1
  measures "d11" radius of A2
  measures "d12" radius of A3
extrude "Extrude1" add sketch "Sketch2" along normal blind 4 contours L0 L1 L2 L3 A0 A1 A2 A3 | S0 L4 S1 S2 S3 S4 S5 S6 S7 S8 S9 L5 S10 S11 L6 S12 S13 S14 S15 S16 S17 S18 S19 S20 L7 S21 S22 S23 S24 L8 S25 L9 S26 L10 S27 S28 S29 S30 S31 L11 S32 L12 S33 S34 S35 S36 S37 S38 L13 S39 S40 S41 S42 L14 S43 S44 S45 S46 S47 S48 S49 S50 L15 S51 S52 S53 L16 S54 L17 L18 S55 S56 S57 S58 S59 S60 S61 S62 S63 S64 S65 S66 S67 S68 S69 S70 S71 S72 S73 L19 S74 S75 L20 S76 S77 S78 S79 L21 S80 L22 S81 S82 L55 | S83 L23 S84 L24 S85 S86 S87 S88 S89 S90 S91 S92 S93 S94 S95 S96 S97 S98 S99 S100 S101 S102 L25 S103 S104 S105 S106 S107 L26 S108 S109 S110 S111 S112 L27 S113 S114 S115 S116 S117 S118 L28 S119 L29 S120 S121 S122 S123 L30 L31 S124 S125 S126 S127 S128 S129 S130 S131 S132 L32 S133 S134 S135 | S136 L33 S137 S138 S139 S140 S141 S142 S143 S144 S145 S146 S147 S148 S149 S150 S151 S152 S153 S154 S155 S156 S157 S158 S159 S160 S161 S162 L34 S163 S164 S165 L35 S166 S167 S168 S169 L36 S170 L37 S171 L38 S172 S173 L39 S174 S175 S176 | S177 S178 L40 S179 S180 S181 S182 S183 S184 S185 S186 L41 S187 S188 S189 S190 L42 S191 L43 S192 L44 S193 S194 S195 S196 S197 S198 L45 S199 S200 S201 S202 S203 S204 S205 S206 S207 S208 S209 S210 S211 S212 S213 S214 S215 L46 S216 S217 L47 S218 S219 S220 S221 L48 S222 L49 S223 S224 | S225 S226 L50 S227 S228 S229 S230 S231 S232 S233 L51 S234 S235 S236 L52 S237 S238 S239 S240 L53 S241 S242 L54 S243 S244 S245 S246 S247 S248 S249 S250 S251 S252 S253 S254 S255 S256 S257 S258 S259 S260 S261 S262 S263 S264 | S265 S266 S267 S268 S269 S270 | S271 S272 S273 S274 S275 S276 makes body 1
extrude "Extrude2" add sketch "Sketch2" along normal blind 7 contours S0 L4 S1 S2 S3 S4 S5 S6 S7 S8 S9 L5 S10 S11 L6 S12 S13 S14 S15 S16 S17 S18 S19 S20 L7 S21 S22 S23 S24 L8 S25 L9 S26 L10 S27 S28 S29 S30 S31 L11 S32 L12 S33 S34 S35 S36 S37 S38 L13 S39 S40 S41 S42 L14 S43 S44 S45 S46 S47 S48 S49 S50 L15 S51 S52 S53 L16 S54 L17 L18 S55 S56 S57 S58 S59 S60 S61 S62 S63 S64 S65 S66 S67 S68 S69 S70 S71 S72 S73 L19 S74 S75 L20 S76 S77 S78 S79 L21 S80 L22 S81 S82 L55 | S83 L23 S84 L24 S85 S86 S87 S88 S89 S90 S91 S92 S93 S94 S95 S96 S97 S98 S99 S100 S101 S102 L25 S103 S104 S105 S106 S107 L26 S108 S109 S110 S111 S112 L27 S113 S114 S115 S116 S117 S118 L28 S119 L29 S120 S121 S122 S123 L30 L31 S124 S125 S126 S127 S128 S129 S130 S131 S132 L32 S133 S134 S135 | S136 L33 S137 S138 S139 S140 S141 S142 S143 S144 S145 S146 S147 S148 S149 S150 S151 S152 S153 S154 S155 S156 S157 S158 S159 S160 S161 S162 L34 S163 S164 S165 L35 S166 S167 S168 S169 L36 S170 L37 S171 L38 S172 S173 L39 S174 S175 S176 | S177 S178 L40 S179 S180 S181 S182 S183 S184 S185 S186 L41 S187 S188 S189 S190 L42 S191 L43 S192 L44 S193 S194 S195 S196 S197 S198 L45 S199 S200 S201 S202 S203 S204 S205 S206 S207 S208 S209 S210 S211 S212 S213 S214 S215 L46 S216 S217 L47 S218 S219 S220 S221 L48 S222 L49 S223 S224 | S225 S226 L50 S227 S228 S229 S230 S231 S232 S233 L51 S234 S235 S236 L52 S237 S238 S239 S240 L53 S241 S242 L54 S243 S244 S245 S246 S247 S248 S249 S250 S251 S252 S253 S254 S255 S256 S257 S258 S259 S260 S261 S262 S263 S264 | S265 S266 S267 S268 S269 S270 | S271 S272 S273 S274 S275 S276 bodies 1
fillet "Fillet2" chord length 1 8 edges at (15, 0, 4) (14.4142, 10.4142, 4) (0, 11, 4) (-14.4142, 10.4142, 4) (-15, 0, 4) (-14.4142, -10.4142, 4) (0, -11, 4) (14.4142, -10.4142, 4) on bodies 1
chamfer "Chamfer1" distance 0.2 angle 45 8 edges at (14.4142, -10.4142, 0) (0, -11, 0) (-14.4142, -10.4142, 0) (-15, 0, 0) (-14.4142, 10.4142, 0) (0, 11, 0) (14.4142, 10.4142, 0) (15, 0, 0) on bodies 1
extrude "Extrude3" add sketch "Sketch2" against normal blind 4 separate body contours L0 L1 L2 L3 A0 A1 A2 A3 | S0 L4 S1 S2 S3 S4 S5 S6 S7 S8 S9 L5 S10 S11 L6 S12 S13 S14 S15 S16 S17 S18 S19 S20 L7 S21 S22 S23 S24 L8 S25 L9 S26 L10 S27 S28 S29 S30 S31 L11 S32 L12 S33 S34 S35 S36 S37 S38 L13 S39 S40 S41 S42 L14 S43 S44 S45 S46 S47 S48 S49 S50 L15 S51 S52 S53 L16 S54 L17 L18 S55 S56 S57 S58 S59 S60 S61 S62 S63 S64 S65 S66 S67 S68 S69 S70 S71 S72 S73 L19 S74 S75 L20 S76 S77 S78 S79 L21 S80 L22 S81 S82 L55 | S83 L23 S84 L24 S85 S86 S87 S88 S89 S90 S91 S92 S93 S94 S95 S96 S97 S98 S99 S100 S101 S102 L25 S103 S104 S105 S106 S107 L26 S108 S109 S110 S111 S112 L27 S113 S114 S115 S116 S117 S118 L28 S119 L29 S120 S121 S122 S123 L30 L31 S124 S125 S126 S127 S128 S129 S130 S131 S132 L32 S133 S134 S135 | S136 L33 S137 S138 S139 S140 S141 S142 S143 S144 S145 S146 S147 S148 S149 S150 S151 S152 S153 S154 S155 S156 S157 S158 S159 S160 S161 S162 L34 S163 S164 S165 L35 S166 S167 S168 S169 L36 S170 L37 S171 L38 S172 S173 L39 S174 S175 S176 | S177 S178 L40 S179 S180 S181 S182 S183 S184 S185 S186 L41 S187 S188 S189 S190 L42 S191 L43 S192 L44 S193 S194 S195 S196 S197 S198 L45 S199 S200 S201 S202 S203 S204 S205 S206 S207 S208 S209 S210 S211 S212 S213 S214 S215 L46 S216 S217 L47 S218 S219 S220 S221 L48 S222 L49 S223 S224 | S225 S226 L50 S227 S228 S229 S230 S231 S232 S233 L51 S234 S235 S236 L52 S237 S238 S239 S240 L53 S241 S242 L54 S243 S244 S245 S246 S247 S248 S249 S250 S251 S252 S253 S254 S255 S256 S257 S258 S259 S260 S261 S262 S263 S264 | S265 S266 S267 S268 S269 S270 | S271 S272 S273 S274 S275 S276 makes body 2
sketch "Sketch3" plane through (0, 0, -4) normal (0, 0, -1) x (1, 0, 0)
  arc A0 (-15, -9) -> (-13, -11) centre (-13, -9) ccw
  line L0 (-13, -11) -> (13, -11)
  arc A1 (13, -11) -> (15, -9) centre (13, -9) ccw
  line L1 (15, -9) -> (15, 9)
  arc A2 (15, 9) -> (13, 11) centre (13, 9) ccw
  line L2 (13, 11) -> (-13, 11)
  arc A3 (-13, 11) -> (-15, 9) centre (-13, 9) ccw
  line L3 (-15, 9) -> (-15, -9)
  line L4 (0, 0) -> (3.8333, 0) construction
  line L5 (0, 0) -> (-3.8333, 0) construction
  line L6 (-3.8333, 0) -> (-11.5, 0) construction
  line L7 (3.8333, 0) -> (11.5, 0) construction
  circle A4 centre (-3.8333, 0) radius 2.5
  circle A5 centre (3.8333, 0) radius 2.5
  circle A6 centre (-11.5, 0) radius 2.5
  circle A7 centre (11.5, 0) radius 2.5
  line L8 (-15, 11) -> (15, 11)
  line L9 (15, 11) -> (15, -11)
  line L10 (15, -11) -> (-15, -11)
  line L11 (-15, -11) -> (-15, 11)
  dimension "d22" = 3.8333
  dimension "d23" = 3.8333
  dimension "d24" = 7.6667
  dimension "d25" = 7.6667
  dimension "d26" = 5
  dimension "d27" = 5
  dimension "d28" = 5
  dimension "d29" = 5
  constraint coincident L4.start L5.start
  constraint horizontal L4
  constraint parallel L4 L5
  constraint parallel L5 L6
  constraint horizontal L7
  constraint coincident L5.end L6.start
  constraint coincident L4.end L7.start
  constraint coincident L6.end A6.centre
  constraint coincident L7.end A7.centre
  constraint horizontal L8
  constraint vertical L9
  constraint horizontal L10
  constraint vertical L11
  measures "d22" distance of L4.start L4.end
  measures "d23" distance of L4.start L5.end
  measures "d24" distance of L5.end L6.end
  measures "d25" distance of L4.end L7.end
  measures "d26" diameter of A4
  measures "d27" diameter of A5
  measures "d28" diameter of A6
  measures "d29" diameter of A7
extrude "Extrude4" cut sketch "Sketch3" against normal blind 2.5 contours A4 | A5 | A6 | A7 bodies 2
copy_body "Body->Comp1" bodies 1 removing the originals makes body 3 in component "TransparentLogo"
copy_body "Body->Comp2" bodies 2 removing the originals makes body 4 in component "Difusor"
component "TransparentLogo" placed x (1, 0, 0) y (0, 1, 0) z (0, 0, 1) at (0, 0, 0)
component "Difusor" placed x (1, 0, 0) y (0, 1, 0) z (0, 0, 1) at (0, 0, 0)
equation "d22 = ( 7.6666 / 2 ) * 1 mm"
equation "d23 = ( 7.6666 / 2 ) * 1 mm"
